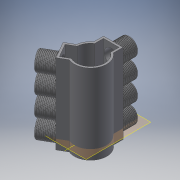
# Autodesk Inventor part: 부품2
Saved by Autodesk Inventor 2018 (Build 220112000, 112)
## iProperties
Created: 2019-05-28
Part Number: 부품2
Material: 일반
Document SubType Name: Modeling
Designer: LeeYounSeo
Mass: 80.4089 g
Surface Area: 542.484 cm^2
Volume: 80.4089 cm^3
Density: 1 g/cm^3
Appearance: 기본값
Author: LeeYounSeo
Autodesk Inventor part; units mm, degrees
ref_plane "YZ Plane" through (0, 0, 0) normal (1, 0, 0) x (0, 1, 0)
ref_plane "XZ Plane" through (0, 0, 0) normal (0, 1, 0) x (-1, 0, 0)
ref_plane "XY Plane" through (0, 0, 0) normal (0, 0, 1) x (1, 0, 0)
sketch "스케치1" plane through (0, 0, 0) normal (0, 0, 1) x (1, 0, 0)
  line L0 (-15, 35) -> (15, 35)
  line L1 (15, 35) -> (15, 20)
  line L2 (-15, 20) -> (-15, 35)
  line L3 (-37.8109, -4.5096) -> (-22.8109, -30.4904)
  line L4 (-22.8109, -30.4904) -> (-9.8205, -22.9904)
  line L5 (-24.8205, 2.9904) -> (-37.8109, -4.5096)
  arc A0 (-9.8205, -22.9904) -> (15, 20) centre (0, 0) ccw
  arc A1 (-15, 20) -> (-24.8205, 2.9904) centre (0, 0) ccw
  point P0 (0, 35)
  dimension "d1" = 30
  dimension "d2" = 15
  dimension "d3" = 120
  dimension "d6" = 30
  dimension "d7" = 15
  constraints: 12 end point, 4 point on circle, 2 centre point, 2 parallel, 2 perpendicular, 1 coincident, 1 horizontal, 1 midpoint, 1 vertical alignment
  measures "d1" distance of L0.start L0.end
  measures "d2" distance of L0.end L1.end
  measures "d3" angle of L2 L5
  measures "d6" distance of L3.start L3.end
  measures "d7" distance of L3.end L4.end
extrude "돌출1" add sketch "스케치1" along normal blind 3
sketch "스케치2" plane through (0, 0, 3) normal (0, 0, 1) x (1, 0, 0)
  point P0 (0, 0)
sketch "스케치3" plane through (0, 0, 3) normal (0, 0, 1) x (1, 0, 0)
  line L0 (15, 35) -> (-15, 35) projected
  line L1 (-15, 35) -> (-15, 20) projected
  arc A0 (-15, 20) -> (-24.8205, 2.9904) centre (0, 0) ccw projected
  line L2 (-24.8205, 2.9904) -> (-37.8109, -4.5096) projected
  line L3 (-37.8109, -4.5096) -> (-22.8109, -30.4904) projected
  line L4 (-22.8109, -30.4904) -> (-9.8205, -22.9904) projected
  arc A1 (-9.8205, -22.9904) -> (15, 20) centre (0, 0) ccw projected
  line L5 (15, 20) -> (15, 35) projected
  arc A2 (-12, 18.4391) -> (-21.9687, 1.1728) centre (0, 0) ccw
  line L6 (-12, 18.4391) -> (-12, 32)
  line L7 (-12, 32) -> (12, 32)
  line L8 (12, 32) -> (12, 18.4391)
  arc A3 (-9.9687, -19.6118) -> (12, 18.4391) centre (0, 0) ccw
  line L9 (-9.9687, -19.6118) -> (-21.7128, -26.3923)
  line L10 (-21.7128, -26.3923) -> (-33.7128, -5.6077)
  line L11 (-33.7128, -5.6077) -> (-21.9687, 1.1728)
  dimension "d10" = 3
  constraints: 12 end point, 4 point on circle, 2 centre point, 7 other
  measures "d10" radial gap between concentric circles of A2 A0
extrude "돌출2" add sketch "스케치3" along normal blind 120
sketch "스케치4" plane through (-15, 35, 0) normal (0, 1, 0) x (1, 0, 0)
  point P0 (15, 0)
sketch "스케치5" plane through (-15, 35, 0) normal (0, 1, 0) x (1, 0, 0)
  line L0 (0, 0) -> (30, 0) projected
  line L1 (0, 0) -> (0, -123) projected
  line L2 (30, -123) -> (0, -123) projected
  line L3 (30, 0) -> (30, -123) projected
  circle A0 centre (15, -15) radius 13.5
  line L4 (0, 0) -> (30, 0) projected
  point P0 (15, 0)
  point P1 (15, 0)
  point P2 (15, 0)
  dimension "d13" = 15
  dimension "d14" = 27
  constraints: 2 midpoint, 2 vertical alignment, 1 centre point
  measures "d13" distance from line of L0 A0.centre
  measures "d14" diameter of A0
extrude "돌출3" add sketch "스케치5" along normal blind 25 contours A0
ref_plane "작업 평면1" through (0, 35, 15) normal (0, 0, 1) x (0, 1, 0)
sketch "스케치6" plane through (0, 35, 15) normal (0, 0, 1) x (0, 1, 0)
  line L0 (0, -13.5) -> (25, -13.5) projected
  line L1 (25, -13.5) -> (25, 13.5) projected
  line L2 (0, 13.5) -> (0, -13.5) projected
  line L3 (0, 13.5) -> (25, 13.5) projected
  line L4 (0, -13.5) -> (1, -13.5)
  line L5 (1, -13.5) -> (1, -12.5)
  line L6 (1, -12.5) -> (0, -12.5)
  line L7 (0, -12.5) -> (0, -13.5)
  line L8 (0, 13.5) -> (0, -13.5) projected
  line L9 (0, 0) -> (11.9782, 0)
  line L10 (-83.5885, 0) -> (43.0981, 0) projected
  point P0 (-35, 0)
  dimension "d18" = 1
  dimension "d19" = 1
  constraints: 10 end point, 2 horizontal, 2 parallel, 1 midpoint, 1 perpendicular
  measures "d18" distance of L4.end L5.end
  measures "d19" distance of L5.end L6.end
revolve "회전1" cut sketch "스케치6" angle 360 about axis through (0, 35, 15) along (0, 1, 0) contours L2 L6 L5 L0
pattern_linear "직사각형 패턴1" count 13 spacing 2 along (0, 1, 0) of "회전1"
sketch "스케치7" plane through (0, 60, 15) normal (0, 1, 0) x (1, 0, 0)
  circle A0 centre (0, 0) radius 12.5 projected
  circle A1 centre (0, 0) radius 12.5 projected
  circle A2 centre (0, 0) radius 12.5 projected
  circle A3 centre (0, 0) radius 11
  point P0 (0, 15)
  dimension "d24" = 22
  constraints: 1 centre point, 1 coincident
  measures "d24" diameter of A3
extrude "돌출4" cut sketch "스케치7" against normal blind 40 contours A3
pattern_circular "원형 패턴1" count 2 over 120 about axis through (0, 0, 0) along (0, 0, 1) of "돌출3", "회전1", "직사각형 패턴1", "돌출4"
pattern_linear "직사각형 패턴2" count 4 spacing 30 along (0, 0, 1) of "돌출3", "회전1", "직사각형 패턴1", "돌출4", "원형 패턴1"
